Autodesk Inventor part; units mm, degrees
(part 2 of 4)
sketch "Sketch20" plane through (0, 0, 1.6) normal (0, 0, 1) x (1, 0, 0)
  line L0 (49, -24.373) -> (49, -33.5) projected
  arc A0 (47, -35.5) -> (49, -33.5) centre (47, -33.5) ccw projected
  line L1 (47, -35.5) -> (37, -35.5) projected
  arc A1 (35, -33.5) -> (37, -35.5) centre (37, -33.5) ccw projected
  line L2 (35, -33.5) -> (35, -24.373) projected
  arc A2 (37, -14.255) -> (35, -24.373) centre (42, -20.5) ccw projected
  line L3 (37, -14.255) -> (37, -6) projected
  arc A3 (47, -6) -> (37, -6) centre (42, -6) ccw projected
  line L4 (47, -6) -> (47, -14.255) projected
  arc A4 (49, -24.373) -> (47, -14.255) centre (42, -20.5) ccw projected
  line L5 (34.5, 22.1) -> (34.5, 39.1) projected
  arc A5 (35.5, 40.1) -> (34.5, 39.1) centre (35.5, 39.1) ccw projected
  line L6 (35.5, 40.1) -> (67.5, 40.1) projected
  arc A6 (68.5, 39.1) -> (67.5, 40.1) centre (67.5, 39.1) ccw projected
  line L7 (68.5, 39.1) -> (68.5, 22.1) projected
  arc A7 (67.5, 21.1) -> (68.5, 22.1) centre (67.5, 22.1) ccw projected
  line L8 (67.5, 21.1) -> (35.5, 21.1) projected
  arc A8 (34.5, 22.1) -> (35.5, 21.1) centre (35.5, 22.1) ccw projected
  circle A9 centre (35.75, 43.95) radius 3 projected
  circle A10 centre (67.25, 43.95) radius 3 projected
  circle A11 centre (67.25, 14.25) radius 3 projected
  circle A12 centre (35.75, 14.25) radius 3 projected
  circle A13 centre (-31.5, -14) radius 3.5 projected
  circle A14 centre (31.5, -14) radius 3.5 projected
  circle A15 centre (-10.5, -14) radius 3.5 projected
  circle A16 centre (10.5, -14) radius 3.5 projected
  line L9 (-47, -33.5) -> (-47, -26.745) projected
  arc A17 (-47, -14.255) -> (-47, -26.745) centre (-42, -20.5) ccw projected
  line L10 (-47, -14.255) -> (-47, -6) projected
  arc A18 (-37, -6) -> (-47, -6) centre (-42, -6) ccw projected
  line L11 (-37, -6) -> (-37, -14.255) projected
  arc A19 (-37, -26.745) -> (-37, -14.255) centre (-42, -20.5) ccw projected
  line L12 (-37, -26.745) -> (-37, -33.5) projected
  arc A20 (-39, -35.5) -> (-37, -33.5) centre (-39, -33.5) ccw projected
  line L13 (-39, -35.5) -> (-45, -35.5) projected
  arc A21 (-47, -33.5) -> (-45, -35.5) centre (-45, -33.5) ccw projected
  line L14 (-26, -33.5) -> (-26, -26.745) projected
  arc A22 (-26, -14.255) -> (-26, -26.745) centre (-21, -20.5) ccw projected
  line L15 (-26, -14.255) -> (-26, -6) projected
  arc A23 (-16, -6) -> (-26, -6) centre (-21, -6) ccw projected
  line L16 (-16, -6) -> (-16, -14.255) projected
  arc A24 (-16, -26.745) -> (-16, -14.255) centre (-21, -20.5) ccw projected
  line L17 (-16, -26.745) -> (-16, -33.5) projected
  arc A25 (-18, -35.5) -> (-16, -33.5) centre (-18, -33.5) ccw projected
  line L18 (-18, -35.5) -> (-24, -35.5) projected
  arc A26 (-26, -33.5) -> (-24, -35.5) centre (-24, -33.5) ccw projected
  line L19 (-5, -33.5) -> (-5, -26.745) projected
  arc A27 (-5, -14.255) -> (-5, -26.745) centre (0, -20.5) ccw projected
  line L20 (-5, -14.255) -> (-5, -6) projected
  arc A28 (5, -6) -> (-5, -6) centre (0, -6) ccw projected
  line L21 (5, -6) -> (5, -14.255) projected
  arc A29 (5, -26.745) -> (5, -14.255) centre (0, -20.5) ccw projected
  line L22 (5, -26.745) -> (5, -33.5) projected
  arc A30 (3, -35.5) -> (5, -33.5) centre (3, -33.5) ccw projected
  line L23 (3, -35.5) -> (-3, -35.5) projected
  arc A31 (-5, -33.5) -> (-3, -35.5) centre (-3, -33.5) ccw projected
  line L24 (16, -33.5) -> (16, -26.745) projected
  arc A32 (16, -14.255) -> (16, -26.745) centre (21, -20.5) ccw projected
  line L25 (16, -14.255) -> (16, -6) projected
  arc A33 (26, -6) -> (16, -6) centre (21, -6) ccw projected
  line L26 (26, -6) -> (26, -14.255) projected
  arc A34 (26, -26.745) -> (26, -14.255) centre (21, -20.5) ccw projected
  line L27 (26, -26.745) -> (26, -33.5) projected
  arc A35 (24, -35.5) -> (26, -33.5) centre (24, -33.5) ccw projected
  line L28 (24, -35.5) -> (18, -35.5) projected
  arc A36 (16, -33.5) -> (18, -35.5) centre (18, -33.5) ccw projected
  arc A37 (58, -6.5) -> (56, -8.5) centre (58, -8.5) ccw projected
  line L29 (58, -6.5) -> (70, -6.5) projected
  line L30 (70, -6.5) -> (70, -10.5) projected
  arc A38 (70, -10.5) -> (70.9655, -12.9138) centre (73.5, -10.5) ccw projected
  arc A39 (55.0345, -12.9138) -> (70.9655, -12.9138) centre (63, -20.5) ccw projected
  arc A40 (55.0345, -12.9138) -> (56, -10.5) centre (52.5, -10.5) ccw projected
  line L31 (56, -10.5) -> (56, -8.5) projected
  arc A41 (-58, -34.5) -> (-56, -32.5) centre (-58, -32.5) ccw projected
  line L32 (-58, -34.5) -> (-70, -34.5) projected
  line L33 (-70, -34.5) -> (-70, -30.5) projected
  arc A42 (-70, -30.5) -> (-70.9655, -28.0862) centre (-73.5, -30.5) ccw projected
  arc A43 (-55.0345, -28.0862) -> (-70.9655, -28.0862) centre (-63, -20.5) ccw projected
  arc A44 (-55.0345, -28.0862) -> (-56, -30.5) centre (-52.5, -30.5) ccw projected
  line L34 (-56, -30.5) -> (-56, -32.5) projected
  line L35 (-53.5, 10) -> (-68.5, 10) projected
  arc A45 (-70.7826, 16.1532) -> (-68.5, 10) centre (-68.5, 13.5) ccw projected
  arc A46 (-70.7826, 16.1532) -> (-70, 17.8589) centre (-72.25, 17.8589) ccw projected
  line L36 (-70, 17.8589) -> (-70, 22) projected
  line L37 (-70, 22) -> (-54, 22) projected
  arc A47 (-52, 20) -> (-54, 22) centre (-54, 20) ccw projected
  line L38 (-52, 20) -> (-52, 17.8589) projected
  arc A48 (-52, 17.8589) -> (-51.2174, 16.1532) centre (-49.75, 17.8589) ccw projected
  arc A49 (-53.5, 10) -> (-51.2174, 16.1532) centre (-53.5, 13.5) ccw projected
  line L39 (-70.5, -37.5) -> (-56.7679, -37.5) projected
  line L40 (-56.7679, -37.5) -> (-55.6132, -39.5) projected
  arc A50 (-55.6132, -41.5) -> (-55.6132, -39.5) centre (-57.3453, -40.5) ccw projected
  line L41 (-55.6132, -41.5) -> (-56.7679, -43.5) projected
  line L42 (-56.7679, -43.5) -> (-70.5, -43.5) projected
  line L43 (-70.5, -43.5) -> (-70.5, -47.4689) projected
  arc A51 (-70.5, -47.4689) -> (-69.0556, -48.3647) centre (-69.5, -47.4689) ccw projected
  arc A52 (-64.3647, -53.0556) -> (-69.0556, -48.3647) centre (-67.5, -51.5) ccw projected
  arc A53 (-64.3647, -53.0556) -> (-63.4689, -54.5) centre (-63.4689, -53.5) ccw projected
  line L44 (-63.4689, -54.5) -> (-47, -54.5) projected
  line L45 (-47, -54.5) -> (-47, -50) projected
  arc A54 (-45, -48) -> (-47, -50) centre (-45, -50) ccw projected
  line L46 (-45, -48) -> (24, -48) projected
  arc A55 (26, -50) -> (24, -48) centre (24, -50) ccw projected
  line L47 (26, -50) -> (26, -54.5) projected
  line L48 (26, -54.5) -> (63.4689, -54.5) projected
  arc A56 (63.4689, -54.5) -> (64.3647, -53.0556) centre (63.4689, -53.5) ccw projected
  arc A57 (69.0556, -48.3647) -> (64.3647, -53.0556) centre (67.5, -51.5) ccw projected
  arc A58 (69.0556, -48.3647) -> (70.5, -47.4689) centre (69.5, -47.4689) ccw projected
  line L49 (70.5, -47.4689) -> (70.5, -43.5) projected
  line L50 (70.5, -43.5) -> (57.2321, -43.5) projected
  line L51 (57.2321, -43.5) -> (58.5311, -41.25) projected
  arc A59 (58.5311, -41.25) -> (58.5311, -39.75) centre (57.2321, -40.5) ccw projected
  line L52 (58.5311, -39.75) -> (57.2321, -37.5) projected
  line L53 (57.2321, -37.5) -> (70.5, -37.5) projected
  line L54 (70.5, -37.5) -> (70.5, -30.5) projected
  arc A60 (71.3276, -28.431) -> (70.5, -30.5) centre (73.5, -30.5) ccw projected
  arc A61 (71.3276, -28.431) -> (71.3276, -12.569) centre (63, -20.5) ccw projected
  arc A62 (70.5, -10.5) -> (71.3276, -12.569) centre (73.5, -10.5) ccw projected
  line L55 (70.5, -10.5) -> (70.5, 9.6199) projected
  arc A63 (71, 10.9428) -> (70.5, 9.6199) centre (72.5, 9.6199) ccw projected
  arc A64 (71, 10.9428) -> (72.25, 14.25) centre (67.25, 14.25) ccw projected
  line L56 (72.25, 14.25) -> (72.25, 43.95) projected
  arc A65 (72.25, 43.95) -> (71, 47.2572) centre (67.25, 43.95) ccw projected
  arc A66 (70.6186, 47.9015) -> (71, 47.2572) centre (72.5, 48.5801) ccw projected
  arc A67 (70.6186, 47.9015) -> (69.194, 48.4372) centre (69.678, 47.5622) ccw projected
  arc A68 (64.3647, 53.0556) -> (69.194, 48.4372) centre (67.5, 51.5) ccw projected
  arc A69 (64.3647, 53.0556) -> (63.4689, 54.5) centre (63.4689, 53.5) ccw projected
  line L57 (63.4689, 54.5) -> (-63.4689, 54.5) projected
  arc A70 (-63.4689, 54.5) -> (-64.3647, 53.0556) centre (-63.4689, 53.5) ccw projected
  arc A71 (-69.0556, 48.3647) -> (-64.3647, 53.0556) centre (-67.5, 51.5) ccw projected
  arc A72 (-69.0556, 48.3647) -> (-70.5, 47.4689) centre (-69.5, 47.4689) ccw projected
  line L58 (-70.5, 47.4689) -> (-70.5, 17.8589) projected
  arc A73 (-71.1087, 16.5323) -> (-70.5, 17.8589) centre (-72.25, 17.8589) ccw projected
  arc A74 (-71.1087, 16.5323) -> (-71.1087, 10.4677) centre (-68.5, 13.5) ccw projected
  arc A75 (-70.5, 9.1411) -> (-71.1087, 10.4677) centre (-72.25, 9.1411) ccw projected
  line L59 (-70.5, 9.1411) -> (-70.5, 3) projected
  line L60 (-70.5, 3) -> (-53.1906, 3) projected
  line L61 (-53.1906, 3) -> (-51.7472, 0.5) projected
  arc A76 (-51.7472, -2.5) -> (-51.7472, 0.5) centre (-54.3453, -1) ccw projected
  line L62 (-51.7472, -2.5) -> (-53.1906, -5) projected
  line L63 (-53.1906, -5) -> (-70.5, -5) projected
  line L64 (-70.5, -5) -> (-70.5, -10.5) projected
  arc A77 (-71.3276, -12.569) -> (-70.5, -10.5) centre (-73.5, -10.5) ccw projected
  arc A78 (-71.3276, -12.569) -> (-71.3276, -28.431) centre (-63, -20.5) ccw projected
  arc A79 (-70.5, -30.5) -> (-71.3276, -28.431) centre (-73.5, -30.5) ccw projected
  line L65 (-70.5, -30.5) -> (-70.5, -37.5) projected
  line L66 (34, 39.1) -> (34, 22.1)
  arc A80 (34, 22.1) -> (35.5, 20.6) centre (35.5, 22.1) ccw
  line L67 (35.5, 20.6) -> (67.5, 20.6)
  arc A81 (67.5, 20.6) -> (69, 22.1) centre (67.5, 22.1) ccw
  line L68 (69, 22.1) -> (69, 39.1)
  arc A82 (69, 39.1) -> (67.5, 40.6) centre (67.5, 39.1) ccw
  line L69 (67.5, 40.6) -> (35.5, 40.6)
  arc A83 (35.5, 40.6) -> (34, 39.1) centre (35.5, 39.1) ccw
  line L70 (33.5, 39.1) -> (33.5, 22.1)
  arc A84 (33.5, 22.1) -> (35.5, 20.1) centre (35.5, 22.1) ccw
  line L71 (35.5, 20.1) -> (67.5, 20.1)
  arc A85 (67.5, 20.1) -> (69.5, 22.1) centre (67.5, 22.1) ccw
  line L72 (69.5, 22.1) -> (69.5, 39.1)
  arc A86 (69.5, 39.1) -> (67.5, 41.1) centre (67.5, 39.1) ccw
  line L73 (67.5, 41.1) -> (35.5, 41.1)
  arc A87 (35.5, 41.1) -> (33.5, 39.1) centre (35.5, 39.1) ccw
  circle A88 centre (35.75, 43.95) radius 4
  circle A89 centre (67.25, 43.95) radius 4
  line L74 (33, 22.1) -> (33, 39.1)
  arc A90 (35.5, 41.6) -> (33, 39.1) centre (35.5, 39.1) ccw
  line L75 (35.5, 41.6) -> (67.5, 41.6)
  arc A91 (70, 39.1) -> (67.5, 41.6) centre (67.5, 39.1) ccw
  line L76 (70, 39.1) -> (70, 22.1)
  arc A92 (67.5, 19.6) -> (70, 22.1) centre (67.5, 22.1) ccw
  line L77 (67.5, 19.6) -> (35.5, 19.6)
  arc A93 (33, 22.1) -> (35.5, 19.6) centre (35.5, 22.1) ccw
  line L78 (32.5, 22.1) -> (32.5, 39.1)
  arc A94 (35.5, 42.1) -> (32.5, 39.1) centre (35.5, 39.1) ccw
  line L79 (35.5, 42.1) -> (67.5, 42.1)
  arc A95 (70.5, 39.1) -> (67.5, 42.1) centre (67.5, 39.1) ccw
  line L80 (70.5, 39.1) -> (70.5, 22.1)
  arc A96 (67.5, 19.1) -> (70.5, 22.1) centre (67.5, 22.1) ccw
  line L81 (67.5, 19.1) -> (35.5, 19.1)
  arc A97 (32.5, 22.1) -> (35.5, 19.1) centre (35.5, 22.1) ccw
  point P0 (0, 0)
  point P1 (65.0643, 40.6)
  point P2 (64.4433, 41.1)
  point P3 (38.5567, 41.1)
  point P4 (37.9357, 40.6)
  point P5 (34.4469, 40.1682)
  point P6 (33.9581, 40.3738)
  point P7 (69.0419, 40.3738)
  point P8 (68.5531, 40.1682)
  point P9 (63.7035, 42.1)
  point P10 (39.2965, 42.1)
  point P11 (38.9869, 41.6)
  point P12 (64.0131, 41.6)
  point P13 (33.5215, 40.6283)
  point P14 (33.1245, 40.9322)
  point P15 (69.8755, 40.9322)
  point P16 (69.4785, 40.6283)
  dimension "d168" = 0.5
  dimension "d169" = 0.5
  dimension "d170" = 8
  dimension "d173" = 0.5
  dimension "d174" = 0.5
  constraints: 32 end point, 32 point on circle, 18 centre point, 2 coincident, 1 equal radius, 28 other
  measures "d168" distance between parallel lines of L5 L66
  measures "d169" distance between parallel lines of L72 L68
  measures "d170" diameter of A88
  measures "d173" distance between parallel lines of L80 L76
  measures "d174" distance between parallel lines of L76 L72
extrude "Extrusion15" add sketch "Sketch20" along normal up to surface (0.005 mm away) contours A83 L66 A80 L67 A81 L68 A82 A89 A86 L72 A85 L71 A84 L70 A87 A88 | A88 L73 A89 L69 | A90 L74 A93 L77 A92 L76 A91 A89 A95 L80 A96 L81 A97 L78 A94 A88 | A88 L79 A89 L75
sketch "Sketch23" plane through (42, -6, 1.605) normal (0, 0, 1) x (1, 0, 0)
  circle A0 centre (0, 0) radius 2.75 projected
  arc A1 (5, 0) -> (-5, 0) centre (0, 0) ccw projected
  line L0 (-5, -8.255) -> (-5, 0) projected
  arc A2 (5, -8.255) -> (-5, -8.255) centre (0, -14.5) ccw projected
  line L1 (5, 0) -> (5, -8.255) projected
  line L2 (0, 0) -> (0, -14.5) construction
  line L3 (-0.5, 0) -> (-0.5, -14.5)
  line L4 (0.5, -14.5) -> (0.5, 0)
  arc A3 (0.5, 0) -> (-0.5, 0) centre (0, 0) ccw
  arc A4 (-0.5, -14.5) -> (0.5, -14.5) centre (0, -14.5) ccw
  arc A5 (-0.5, -4.0389) -> (-1.4474, -2.3383) centre (-2.5, -4.0389) ccw
  arc A6 (1.4474, -2.3383) -> (0.5, -4.0389) centre (2.5, -4.0389) ccw
  circle A7 centre (0, 0) radius 2.75 projected
  line L5 (0, 0) -> (0, -24) construction
  line L6 (5, -29.5) -> (-5, -29.5) projected
  line L7 (4.5, 0) -> (4.5, -24)
  line L8 (-4.5, -24) -> (-4.5, 0)
  arc A8 (4.5, 0) -> (-4.5, 0) centre (0, 0) ccw
  arc A9 (-4.5, -24) -> (4.5, -24) centre (0, -24) ccw
  line L9 (-4, 0) -> (-4, -24)
  arc A10 (-4, -24) -> (4, -24) centre (0, -24) ccw
  line L10 (4, -24) -> (4, 0)
  arc A11 (4, 0) -> (-4, 0) centre (0, 0) ccw
  line L11 (-4.5, -24) -> (4.5, -24)
  arc A12 (-7, -18.373) -> (7, -18.373) centre (0, -14.5) ccw projected
  point P0 (-42, 6)
  point P1 (0, -7.25)
  point P2 (-0.5, -6.5156)
  point P3 (0.5, -6.5156)
  point P4 (0.5, -2.7042)
  point P5 (-0.5, -2.7042)
  point P6 (0, -12)
  point P7 (-4.5, -7.8856)
  point P8 (-4, -7.5718)
  point P9 (4, -7.5718)
  point P10 (4.5, -7.8856)
  point P11 (4.5, -21.1144)
  point P12 (4, -21.4282)
  point P13 (4, -24)
  point P14 (-4, -21.4282)
  point P15 (-4.5, -21.1144)
  point P16 (-4, -24)
  dimension "d188" = 1
  dimension "d189" = 2
  dimension "d192" = 0.5
  dimension "d193" = 0.5
  dimension "d194" = 5.5
  constraints: 22 end point, 18 point on circle, 12 tangent, 8 centre point, 3 parallel, 2 midpoint, 2 point on line, 1 equal radius, 1 horizontal, 1 perpendicular, 1 vertical, 3 other
  measures "d188" diameter of A4
  measures "d189" radius of A6
  measures "d192" radial gap between concentric circles of A8 A1
  measures "d193" radial gap between concentric circles of A11 A8
  measures "d194" distance between parallel lines of L6 L11
extrude "Extrusion18" add sketch "Sketch23" along normal up to surface (0.005 mm away) contours A2 L8 A8 L7 L10 A11 L9 | L9 L11 L8 A12 | A12 L7 L11 L10
sketch "Sketch24" plane through (0, 0, 1.6) normal (0, 0, 1) x (1, 0, 0)
  line L0 (33.5, 22.1) -> (33.5, 39.1) projected
  arc A0 (33.9581, 40.3738) -> (33.5, 39.1) centre (35.5, 39.1) ccw projected
  arc A1 (33.9581, 40.3738) -> (34.4469, 40.1682) centre (35.75, 43.95) ccw projected
  arc A2 (34.4469, 40.1682) -> (34, 39.1) centre (35.5, 39.1) ccw projected
  line L1 (34, 39.1) -> (34, 22.1) projected
  arc A3 (34, 22.1) -> (35.5, 20.6) centre (35.5, 22.1) ccw projected
  line L2 (35.5, 20.6) -> (67.5, 20.6) projected
  arc A4 (67.5, 20.6) -> (69, 22.1) centre (67.5, 22.1) ccw projected
  line L3 (69, 22.1) -> (69, 39.1) projected
  arc A5 (69, 39.1) -> (68.5531, 40.1682) centre (67.5, 39.1) ccw projected
  arc A6 (68.5531, 40.1682) -> (69.0419, 40.3738) centre (67.25, 43.95) ccw projected
  arc A7 (69.5, 39.1) -> (69.0419, 40.3738) centre (67.5, 39.1) ccw projected
  line L4 (69.5, 39.1) -> (69.5, 22.1) projected
  arc A8 (67.5, 20.1) -> (69.5, 22.1) centre (67.5, 22.1) ccw projected
  line L5 (67.5, 20.1) -> (35.5, 20.1) projected
  arc A9 (33.5, 22.1) -> (35.5, 20.1) centre (35.5, 22.1) ccw projected
  arc A10 (70.5, 39.1) -> (69.8755, 40.9322) centre (67.5, 39.1) ccw projected
  line L6 (70.5, 39.1) -> (70.5, 22.1) projected
  arc A11 (67.5, 19.1) -> (70.5, 22.1) centre (67.5, 22.1) ccw projected
  line L7 (67.5, 19.1) -> (35.5, 19.1) projected
  arc A12 (32.5, 22.1) -> (35.5, 19.1) centre (35.5, 22.1) ccw projected
  line L8 (32.5, 22.1) -> (32.5, 39.1) projected
  arc A13 (33.1245, 40.9322) -> (32.5, 39.1) centre (35.5, 39.1) ccw projected
  arc A14 (33.1245, 40.9322) -> (33.5215, 40.6283) centre (35.75, 43.95) ccw projected
  arc A15 (33.5215, 40.6283) -> (33, 39.1) centre (35.5, 39.1) ccw projected
  line L9 (33, 39.1) -> (33, 22.1) projected
  arc A16 (33, 22.1) -> (35.5, 19.6) centre (35.5, 22.1) ccw projected
  line L10 (35.5, 19.6) -> (67.5, 19.6) projected
  arc A17 (67.5, 19.6) -> (70, 22.1) centre (67.5, 22.1) ccw projected
  line L11 (70, 22.1) -> (70, 39.1) projected
  arc A18 (70, 39.1) -> (69.4785, 40.6283) centre (67.5, 39.1) ccw projected
  arc A19 (69.4785, 40.6283) -> (69.8755, 40.9322) centre (67.25, 43.95) ccw projected
  arc A20 (37.9357, 40.6) -> (38.5567, 41.1) centre (35.75, 43.95) ccw projected
  line L12 (38.5567, 41.1) -> (64.4433, 41.1) projected
  arc A21 (64.4433, 41.1) -> (65.0643, 40.6) centre (67.25, 43.95) ccw projected
  line L13 (65.0643, 40.6) -> (37.9357, 40.6) projected
  arc A22 (63.7035, 42.1) -> (64.0131, 41.6) centre (67.25, 43.95) ccw projected
  line L14 (64.0131, 41.6) -> (38.9869, 41.6) projected
  arc A23 (38.9869, 41.6) -> (39.2965, 42.1) centre (35.75, 43.95) ccw projected
  line L15 (39.2965, 42.1) -> (63.7035, 42.1) projected
  line L16 (49, -24.373) -> (49, -33.5) projected
  arc A24 (47, -35.5) -> (49, -33.5) centre (47, -33.5) ccw projected
  line L17 (47, -35.5) -> (37, -35.5) projected
  arc A25 (35, -33.5) -> (37, -35.5) centre (37, -33.5) ccw projected
  line L18 (35, -33.5) -> (35, -24.373) projected
  arc A26 (37, -14.255) -> (35, -24.373) centre (42, -20.5) ccw projected
  line L19 (37, -14.255) -> (37, -6) projected
  arc A27 (47, -6) -> (37, -6) centre (42, -6) ccw projected
  line L20 (47, -6) -> (47, -14.255) projected
  arc A28 (49, -24.373) -> (47, -14.255) centre (42, -20.5) ccw projected
  line L21 (34.5, 22.1) -> (34.5, 39.1) projected
  arc A29 (35.5, 40.1) -> (34.5, 39.1) centre (35.5, 39.1) ccw projected
  line L22 (35.5, 40.1) -> (67.5, 40.1) projected
  arc A30 (68.5, 39.1) -> (67.5, 40.1) centre (67.5, 39.1) ccw projected
  line L23 (68.5, 39.1) -> (68.5, 22.1) projected
  arc A31 (67.5, 21.1) -> (68.5, 22.1) centre (67.5, 22.1) ccw projected
  line L24 (67.5, 21.1) -> (35.5, 21.1) projected
  arc A32 (34.5, 22.1) -> (35.5, 21.1) centre (35.5, 22.1) ccw projected
  circle A33 centre (35.75, 43.95) radius 3 projected
  circle A34 centre (67.25, 43.95) radius 3 projected
  circle A35 centre (67.25, 14.25) radius 3 projected
  circle A36 centre (35.75, 14.25) radius 3 projected
  circle A37 centre (-31.5, -14) radius 3.5 projected
  circle A38 centre (31.5, -14) radius 3.5 projected
  circle A39 centre (-10.5, -14) radius 3.5 projected
  circle A40 centre (10.5, -14) radius 3.5 projected
  line L25 (-47, -33.5) -> (-47, -26.745) projected
  arc A41 (-47, -14.255) -> (-47, -26.745) centre (-42, -20.5) ccw projected
  line L26 (-47, -14.255) -> (-47, -6) projected
  arc A42 (-37, -6) -> (-47, -6) centre (-42, -6) ccw projected
  line L27 (-37, -6) -> (-37, -14.255) projected
  arc A43 (-37, -26.745) -> (-37, -14.255) centre (-42, -20.5) ccw projected
  line L28 (-37, -26.745) -> (-37, -33.5) projected
  arc A44 (-39, -35.5) -> (-37, -33.5) centre (-39, -33.5) ccw projected
  line L29 (-39, -35.5) -> (-45, -35.5) projected
  arc A45 (-47, -33.5) -> (-45, -35.5) centre (-45, -33.5) ccw projected
  line L30 (-26, -33.5) -> (-26, -26.745) projected
  arc A46 (-26, -14.255) -> (-26, -26.745) centre (-21, -20.5) ccw projected
  line L31 (-26, -14.255) -> (-26, -6) projected
  arc A47 (-16, -6) -> (-26, -6) centre (-21, -6) ccw projected
  line L32 (-16, -6) -> (-16, -14.255) projected
  arc A48 (-16, -26.745) -> (-16, -14.255) centre (-21, -20.5) ccw projected
  line L33 (-16, -26.745) -> (-16, -33.5) projected
  arc A49 (-18, -35.5) -> (-16, -33.5) centre (-18, -33.5) ccw projected
  line L34 (-18, -35.5) -> (-24, -35.5) projected
  arc A50 (-26, -33.5) -> (-24, -35.5) centre (-24, -33.5) ccw projected
  line L35 (-5, -33.5) -> (-5, -26.745) projected
  arc A51 (-5, -14.255) -> (-5, -26.745) centre (0, -20.5) ccw projected
  line L36 (-5, -14.255) -> (-5, -6) projected
  arc A52 (5, -6) -> (-5, -6) centre (0, -6) ccw projected
  line L37 (5, -6) -> (5, -14.255) projected
  arc A53 (5, -26.745) -> (5, -14.255) centre (0, -20.5) ccw projected
  line L38 (5, -26.745) -> (5, -33.5) projected
  arc A54 (3, -35.5) -> (5, -33.5) centre (3, -33.5) ccw projected
  line L39 (3, -35.5) -> (-3, -35.5) projected
  arc A55 (-5, -33.5) -> (-3, -35.5) centre (-3, -33.5) ccw projected
  line L40 (16, -33.5) -> (16, -26.745) projected
  arc A56 (16, -14.255) -> (16, -26.745) centre (21, -20.5) ccw projected
  line L41 (16, -14.255) -> (16, -6) projected
  arc A57 (26, -6) -> (16, -6) centre (21, -6) ccw projected
  line L42 (26, -6) -> (26, -14.255) projected
  arc A58 (26, -26.745) -> (26, -14.255) centre (21, -20.5) ccw projected
  line L43 (26, -26.745) -> (26, -33.5) projected
  arc A59 (24, -35.5) -> (26, -33.5) centre (24, -33.5) ccw projected
  line L44 (24, -35.5) -> (18, -35.5) projected
  arc A60 (16, -33.5) -> (18, -35.5) centre (18, -33.5) ccw projected
  arc A61 (58, -6.5) -> (56, -8.5) centre (58, -8.5) ccw projected
  line L45 (58, -6.5) -> (70, -6.5) projected
  line L46 (70, -6.5) -> (70, -10.5) projected
  arc A62 (70, -10.5) -> (70.9655, -12.9138) centre (73.5, -10.5) ccw projected
  arc A63 (55.0345, -12.9138) -> (70.9655, -12.9138) centre (63, -20.5) ccw projected
  arc A64 (55.0345, -12.9138) -> (56, -10.5) centre (52.5, -10.5) ccw projected
  line L47 (56, -10.5) -> (56, -8.5) projected
  arc A65 (-58, -34.5) -> (-56, -32.5) centre (-58, -32.5) ccw projected
  line L48 (-58, -34.5) -> (-70, -34.5) projected
  line L49 (-70, -34.5) -> (-70, -30.5) projected
  arc A66 (-70, -30.5) -> (-70.9655, -28.0862) centre (-73.5, -30.5) ccw projected
  arc A67 (-55.0345, -28.0862) -> (-70.9655, -28.0862) centre (-63, -20.5) ccw projected
  arc A68 (-55.0345, -28.0862) -> (-56, -30.5) centre (-52.5, -30.5) ccw projected
  line L50 (-56, -30.5) -> (-56, -32.5) projected
  line L51 (-53.5, 10) -> (-68.5, 10) projected
  arc A69 (-70.7826, 16.1532) -> (-68.5, 10) centre (-68.5, 13.5) ccw projected
  arc A70 (-70.7826, 16.1532) -> (-70, 17.8589) centre (-72.25, 17.8589) ccw projected
  line L52 (-70, 17.8589) -> (-70, 22) projected
  line L53 (-70, 22) -> (-54, 22) projected
  arc A71 (-52, 20) -> (-54, 22) centre (-54, 20) ccw projected
  line L54 (-52, 20) -> (-52, 17.8589) projected
  arc A72 (-52, 17.8589) -> (-51.2174, 16.1532) centre (-49.75, 17.8589) ccw projected
  arc A73 (-53.5, 10) -> (-51.2174, 16.1532) centre (-53.5, 13.5) ccw projected
  line L55 (-70.5, -37.5) -> (-56.7679, -37.5) projected
  line L56 (-56.7679, -37.5) -> (-55.6132, -39.5) projected
  arc A74 (-55.6132, -41.5) -> (-55.6132, -39.5) centre (-57.3453, -40.5) ccw projected
  line L57 (-55.6132, -41.5) -> (-56.7679, -43.5) projected
  line L58 (-56.7679, -43.5) -> (-70.5, -43.5) projected
  line L59 (-70.5, -43.5) -> (-70.5, -47.4689) projected
  arc A75 (-70.5, -47.4689) -> (-69.0556, -48.3647) centre (-69.5, -47.4689) ccw projected
  arc A76 (-64.3647, -53.0556) -> (-69.0556, -48.3647) centre (-67.5, -51.5) ccw projected
  arc A77 (-64.3647, -53.0556) -> (-63.4689, -54.5) centre (-63.4689, -53.5) ccw projected
  line L60 (-63.4689, -54.5) -> (-47, -54.5) projected
  line L61 (-47, -54.5) -> (-47, -50) projected
  arc A78 (-45, -48) -> (-47, -50) centre (-45, -50) ccw projected
  line L62 (-45, -48) -> (24, -48) projected
  arc A79 (26, -50) -> (24, -48) centre (24, -50) ccw projected
  line L63 (26, -50) -> (26, -54.5) projected
  line L64 (26, -54.5) -> (63.4689, -54.5) projected
  arc A80 (63.4689, -54.5) -> (64.3647, -53.0556) centre (63.4689, -53.5) ccw projected
  arc A81 (69.0556, -48.3647) -> (64.3647, -53.0556) centre (67.5, -51.5) ccw projected
  arc A82 (69.0556, -48.3647) -> (70.5, -47.4689) centre (69.5, -47.4689) ccw projected
  line L65 (70.5, -47.4689) -> (70.5, -43.5) projected
  line L66 (70.5, -43.5) -> (57.2321, -43.5) projected
  line L67 (57.2321, -43.5) -> (58.5311, -41.25) projected
  arc A83 (58.5311, -41.25) -> (58.5311, -39.75) centre (57.2321, -40.5) ccw projected
  line L68 (58.5311, -39.75) -> (57.2321, -37.5) projected
  line L69 (57.2321, -37.5) -> (70.5, -37.5) projected
  line L70 (70.5, -37.5) -> (70.5, -30.5) projected
  arc A84 (71.3276, -28.431) -> (70.5, -30.5) centre (73.5, -30.5) ccw projected
  arc A85 (71.3276, -28.431) -> (71.3276, -12.569) centre (63, -20.5) ccw projected
  arc A86 (70.5, -10.5) -> (71.3276, -12.569) centre (73.5, -10.5) ccw projected
  line L71 (70.5, -10.5) -> (70.5, 9.6199) projected
  arc A87 (71, 10.9428) -> (70.5, 9.6199) centre (72.5, 9.6199) ccw projected
  arc A88 (71, 10.9428) -> (72.25, 14.25) centre (67.25, 14.25) ccw projected
  line L72 (72.25, 14.25) -> (72.25, 43.95) projected
  arc A89 (72.25, 43.95) -> (71, 47.2572) centre (67.25, 43.95) ccw projected
  arc A90 (70.6186, 47.9015) -> (71, 47.2572) centre (72.5, 48.5801) ccw projected
  arc A91 (70.6186, 47.9015) -> (69.194, 48.4372) centre (69.678, 47.5622) ccw projected
  arc A92 (64.3647, 53.0556) -> (69.194, 48.4372) centre (67.5, 51.5) ccw projected
  arc A93 (64.3647, 53.0556) -> (63.4689, 54.5) centre (63.4689, 53.5) ccw projected
  line L73 (63.4689, 54.5) -> (-63.4689, 54.5) projected
  arc A94 (-63.4689, 54.5) -> (-64.3647, 53.0556) centre (-63.4689, 53.5) ccw projected
  arc A95 (-69.0556, 48.3647) -> (-64.3647, 53.0556) centre (-67.5, 51.5) ccw projected
  arc A96 (-69.0556, 48.3647) -> (-70.5, 47.4689) centre (-69.5, 47.4689) ccw projected
  line L74 (-70.5, 47.4689) -> (-70.5, 17.8589) projected
  arc A97 (-71.1087, 16.5323) -> (-70.5, 17.8589) centre (-72.25, 17.8589) ccw projected
  arc A98 (-71.1087, 16.5323) -> (-71.1087, 10.4677) centre (-68.5, 13.5) ccw projected
  arc A99 (-70.5, 9.1411) -> (-71.1087, 10.4677) centre (-72.25, 9.1411) ccw projected
  line L75 (-70.5, 9.1411) -> (-70.5, 3) projected
  line L76 (-70.5, 3) -> (-53.1906, 3) projected
  line L77 (-53.1906, 3) -> (-51.7472, 0.5) projected
  arc A100 (-51.7472, -2.5) -> (-51.7472, 0.5) centre (-54.3453, -1) ccw projected
  line L78 (-51.7472, -2.5) -> (-53.1906, -5) projected
  line L79 (-53.1906, -5) -> (-70.5, -5) projected
  line L80 (-70.5, -5) -> (-70.5, -10.5) projected
  arc A101 (-71.3276, -12.569) -> (-70.5, -10.5) centre (-73.5, -10.5) ccw projected
  arc A102 (-71.3276, -12.569) -> (-71.3276, -28.431) centre (-63, -20.5) ccw projected
  arc A103 (-70.5, -30.5) -> (-71.3276, -28.431) centre (-73.5, -30.5) ccw projected
  line L81 (-70.5, -30.5) -> (-70.5, -37.5) projected
  line L82 (-63.4689, 54) -> (63.4689, 54)
  arc A104 (63.9168, 53.2778) -> (63.4689, 54) centre (63.4689, 53.5) ccw
  arc A105 (63.9168, 53.2778) -> (69.436, 47.9997) centre (67.5, 51.5) ccw
  arc A106 (70.1483, 47.7318) -> (69.436, 47.9997) centre (69.678, 47.5622) ccw
  arc A107 (70.1483, 47.7318) -> (70.625, 46.9265) centre (72.5, 48.5801) ccw
  arc A108 (71.75, 43.95) -> (70.625, 46.9265) centre (67.25, 43.95) ccw
  line L83 (71.75, 43.95) -> (71.75, 14.25)
  arc A109 (70.625, 11.2735) -> (71.75, 14.25) centre (67.25, 14.25) ccw
  arc A110 (70.625, 11.2735) -> (70, 9.6199) centre (72.5, 9.6199) ccw
  line L84 (70, 9.6199) -> (70, -10.5)
  arc A111 (70, -10.5) -> (70.9655, -12.9138) centre (73.5, -10.5) ccw
  arc A112 (70.9655, -28.0862) -> (70.9655, -12.9138) centre (63, -20.5) ccw
  arc A113 (70.9655, -28.0862) -> (70, -30.5) centre (73.5, -30.5) ccw
  line L85 (70, -30.5) -> (70, -37)
  line L86 (70, -37) -> (56.366, -37)
  line L87 (56.366, -37) -> (58.0981, -40)
  arc A114 (58.0981, -41) -> (58.0981, -40) centre (57.2321, -40.5) ccw
  line L88 (58.0981, -41) -> (56.366, -44)
  line L89 (56.366, -44) -> (70, -44)
  line L90 (70, -44) -> (70, -47.4689)
  arc A115 (69.2778, -47.9168) -> (70, -47.4689) centre (69.5, -47.4689) ccw
  arc A116 (69.2778, -47.9168) -> (63.9168, -53.2778) centre (67.5, -51.5) ccw
  arc A117 (63.4689, -54) -> (63.9168, -53.2778) centre (63.4689, -53.5) ccw
  line L91 (63.4689, -54) -> (26.5, -54)
  line L92 (26.5, -54) -> (26.5, -50)
  arc A118 (26.5, -50) -> (24, -47.5) centre (24, -50) ccw
  line L93 (24, -47.5) -> (-45, -47.5)
  arc A119 (-45, -47.5) -> (-47.5, -50) centre (-45, -50) ccw
  line L94 (-47.5, -50) -> (-47.5, -54)
  line L95 (-47.5, -54) -> (-63.4689, -54)
  arc A120 (-63.9168, -53.2778) -> (-63.4689, -54) centre (-63.4689, -53.5) ccw
  arc A121 (-63.9168, -53.2778) -> (-69.2778, -47.9168) centre (-67.5, -51.5) ccw
  arc A122 (-70, -47.4689) -> (-69.2778, -47.9168) centre (-69.5, -47.4689) ccw
  line L96 (-70, -47.4689) -> (-70, -44)
  line L97 (-70, -44) -> (-56.4793, -44)
  line L98 (-56.4793, -44) -> (-55.1802, -41.75)
  arc A123 (-55.1802, -41.75) -> (-55.1802, -39.25) centre (-57.3453, -40.5) ccw
  line L99 (-55.1802, -39.25) -> (-56.4793, -37)
  line L100 (-56.4793, -37) -> (-70, -37)
  line L101 (-70, -37) -> (-70, -30.5)
  arc A124 (-70, -30.5) -> (-70.9655, -28.0862) centre (-73.5, -30.5) ccw
  arc A125 (-70.9655, -12.9138) -> (-70.9655, -28.0862) centre (-63, -20.5) ccw
  arc A126 (-70.9655, -12.9138) -> (-70, -10.5) centre (-73.5, -10.5) ccw
  line L102 (-70, -10.5) -> (-70, -5.5)
  line L103 (-70, -5.5) -> (-52.9019, -5.5)
  line L104 (-52.9019, -5.5) -> (-51.3142, -2.75)
  arc A127 (-51.3142, -2.75) -> (-51.3142, 0.75) centre (-54.3453, -1) ccw
  line L105 (-51.3142, 0.75) -> (-52.9019, 3.5)
  line L106 (-52.9019, 3.5) -> (-70, 3.5)
  line L107 (-70, 3.5) -> (-70, 9.1411)
  arc A128 (-70, 9.1411) -> (-70.7826, 10.8468) centre (-72.25, 9.1411) ccw
  arc A129 (-70.7826, 16.1532) -> (-70.7826, 10.8468) centre (-68.5, 13.5) ccw
  arc A130 (-70.7826, 16.1532) -> (-70, 17.8589) centre (-72.25, 17.8589) ccw
  line L108 (-70, 17.8589) -> (-70, 47.4689)
  arc A131 (-69.2778, 47.9168) -> (-70, 47.4689) centre (-69.5, 47.4689) ccw
  arc A132 (-69.2778, 47.9168) -> (-63.9168, 53.2778) centre (-67.5, 51.5) ccw
  arc A133 (-63.4689, 54) -> (-63.9168, 53.2778) centre (-63.4689, 53.5) ccw
  arc A134 (70.5, -10.5) -> (71.3276, -12.569) centre (73.5, -10.5) ccw
  line L109 (70.5, -10.5) -> (70.5, -6)
  line L110 (70.5, -6) -> (58, -6)
  arc A135 (58, -6) -> (55.5, -8.5) centre (58, -8.5) ccw
  line L111 (55.5, -8.5) -> (55.5, -10.5)
  arc A136 (54.6724, -12.569) -> (55.5, -10.5) centre (52.5, -10.5) ccw
  arc A137 (54.6724, -12.569) -> (71.3276, -12.569) centre (63, -20.5) ccw
  line L112 (47.5, -14.0193) -> (47.5, -6)
  arc A138 (47.5, -6) -> (36.5, -6) centre (42, -6) ccw
  line L113 (36.5, -6) -> (36.5, -14.0193)
  arc A139 (36.5, -14.0193) -> (34.5, -24.5) centre (42, -20.5) ccw
  line L114 (34.5, -24.5) -> (34.5, -33.5)
  arc A140 (34.5, -33.5) -> (37, -36) centre (37, -33.5) ccw
  line L115 (37, -36) -> (47, -36)
  arc A141 (47, -36) -> (49.5, -33.5) centre (47, -33.5) ccw
  line L116 (49.5, -33.5) -> (49.5, -24.5)
  arc A142 (49.5, -24.5) -> (47.5, -14.0193) centre (42, -20.5) ccw
  circle A143 centre (31.5, -14) radius 4
  line L117 (26.5, -14.0193) -> (26.5, -6)
  arc A144 (26.5, -6) -> (15.5, -6) centre (21, -6) ccw
  line L118 (15.5, -6) -> (15.5, -14.0193)
  arc A145 (15.5, -14.0193) -> (15.5, -26.9807) centre (21, -20.5) ccw
  line L119 (15.5, -26.9807) -> (15.5, -33.5)
  arc A146 (15.5, -33.5) -> (18, -36) centre (18, -33.5) ccw
  line L120 (18, -36) -> (24, -36)
  arc A147 (24, -36) -> (26.5, -33.5) centre (24, -33.5) ccw
  line L121 (26.5, -33.5) -> (26.5, -26.9807)
  arc A148 (26.5, -26.9807) -> (26.5, -14.0193) centre (21, -20.5) ccw
  line L122 (5.5, -14.0193) -> (5.5, -6)
  arc A149 (5.5, -6) -> (-5.5, -6) centre (0, -6) ccw
  line L123 (-5.5, -6) -> (-5.5, -14.0193)
  arc A150 (-5.5, -14.0193) -> (-5.5, -26.9807) centre (0, -20.5) ccw
  line L124 (-5.5, -26.9807) -> (-5.5, -33.5)
  arc A151 (-5.5, -33.5) -> (-3, -36) centre (-3, -33.5) ccw
  line L125 (-3, -36) -> (3, -36)
  arc A152 (3, -36) -> (5.5, -33.5) centre (3, -33.5) ccw
  line L126 (5.5, -33.5) -> (5.5, -26.9807)
  arc A153 (5.5, -26.9807) -> (5.5, -14.0193) centre (0, -20.5) ccw
  circle A154 centre (10.5, -14) radius 4
  circle A155 centre (-10.5, -14) radius 4
  line L127 (-15.5, -14.0193) -> (-15.5, -6)
  arc A156 (-15.5, -6) -> (-26.5, -6) centre (-21, -6) ccw
  line L128 (-26.5, -6) -> (-26.5, -14.0193)
  arc A157 (-26.5, -14.0193) -> (-26.5, -26.9807) centre (-21, -20.5) ccw
  line L129 (-26.5, -26.9807) -> (-26.5, -33.5)
  arc A158 (-26.5, -33.5) -> (-24, -36) centre (-24, -33.5) ccw
  line L130 (-24, -36) -> (-18, -36)
  arc A159 (-18, -36) -> (-15.5, -33.5) centre (-18, -33.5) ccw
  line L131 (-15.5, -33.5) -> (-15.5, -26.9807)
  arc A160 (-15.5, -26.9807) -> (-15.5, -14.0193) centre (-21, -20.5) ccw
  circle A161 centre (-31.5, -14) radius 4
  line L132 (-36.5, -14.0193) -> (-36.5, -6)
  arc A162 (-36.5, -6) -> (-47.5, -6) centre (-42, -6) ccw
  line L133 (-47.5, -6) -> (-47.5, -14.0193)
  arc A163 (-47.5, -14.0193) -> (-47.5, -26.9807) centre (-42, -20.5) ccw
  line L134 (-47.5, -26.9807) -> (-47.5, -33.5)
  arc A164 (-47.5, -33.5) -> (-45, -36) centre (-45, -33.5) ccw
  line L135 (-45, -36) -> (-39, -36)
  arc A165 (-39, -36) -> (-36.5, -33.5) centre (-39, -33.5) ccw
  line L136 (-36.5, -33.5) -> (-36.5, -26.9807)
  arc A166 (-36.5, -26.9807) -> (-36.5, -14.0193) centre (-42, -20.5) ccw
  arc A167 (-70.5, -30.5) -> (-71.3276, -28.431) centre (-73.5, -30.5) ccw
  line L137 (-70.5, -30.5) -> (-70.5, -35)
  line L138 (-70.5, -35) -> (-58, -35)
  arc A168 (-58, -35) -> (-55.5, -32.5) centre (-58, -32.5) ccw
  line L139 (-55.5, -32.5) -> (-55.5, -30.5)
  arc A169 (-54.6724, -28.431) -> (-55.5, -30.5) centre (-52.5, -30.5) ccw
  arc A170 (-54.6724, -28.431) -> (-71.3276, -28.431) centre (-63, -20.5) ccw
  line L140 (-54, 22.5) -> (-70.5, 22.5)
  line L141 (-70.5, 22.5) -> (-70.5, 17.8589)
  arc A171 (-71.1087, 16.5323) -> (-70.5, 17.8589) centre (-72.25, 17.8589) ccw
  arc A172 (-71.1087, 16.5323) -> (-68.5, 9.5) centre (-68.5, 13.5) ccw
  line L142 (-68.5, 9.5) -> (-53.5, 9.5)
  arc A173 (-53.5, 9.5) -> (-50.8913, 16.5323) centre (-53.5, 13.5) ccw
  arc A174 (-51.5, 17.8589) -> (-50.8913, 16.5323) centre (-49.75, 17.8589) ccw
  line L143 (-51.5, 17.8589) -> (-51.5, 20)
  arc A175 (-51.5, 20) -> (-54, 22.5) centre (-54, 20) ccw
  line L144 (32, 39.1) -> (32, 22.1)
  arc A176 (32, 22.1) -> (35.5, 18.6) centre (35.5, 22.1) ccw
  line L145 (35.5, 18.6) -> (67.5, 18.6)
  arc A177 (67.5, 18.6) -> (71, 22.1) centre (67.5, 22.1) ccw
  line L146 (71, 22.1) -> (71, 39.1)
  arc A178 (71, 39.1) -> (67.5, 42.6) centre (67.5, 39.1) ccw
  line L147 (67.5, 42.6) -> (35.5, 42.6)
  arc A179 (35.5, 42.6) -> (32, 39.1) centre (35.5, 39.1) ccw
  point P0 (0, 0)
  point P1 (-70, 22.5)
  point P2 (-70.1109, 9.8387)
  point P3 (-70.1419, -11.4865)
  point P4 (-70, -35)
  point P5 (70.1419, -29.5135)
  point P6 (70, -6)
  point P7 (34.3389, -16.8179)
  point P8 (28.6611, -16.8179)
  point P9 (13.3389, -16.8179)
  point P10 (7.6611, -16.8179)
  point P11 (-7.6611, -16.8179)
  point P12 (-13.3389, -16.8179)
  point P13 (-28.6611, -16.8179)
  point P14 (-34.3389, -16.8179)
  point P15 (-35.2881, -15.2846)
  point P16 (-27.7119, -15.2846)
  point P17 (-14.2881, -15.2846)
  point P18 (-6.7119, -15.2846)
  point P19 (6.7119, -15.2846)
  point P20 (14.2881, -15.2846)
  point P21 (27.7119, -15.2846)
  point P22 (35.2881, -15.2846)
  point P23 (33.4964, 41.9698)
  point P24 (38.4291, 42.6)
  point P25 (64.5709, 42.6)
  point P26 (69.5036, 41.9698)
  dimension "d195" = 0.5
  dimension "d196" = 0.5
  dimension "d197" = 0.5
  dimension "d198" = 0.5
  dimension "d199" = 0.5
  dimension "d200" = 0.5
  dimension "d201" = 0.5
  dimension "d202" = 0.5
  dimension "d203" = 0.5
  dimension "d204" = 0.5
  dimension "d205" = 0.5
  dimension "d206" = 0.5
  dimension "d207" = 0.5
  dimension "d208" = 0.5
  constraints: 144 point on circle, 132 end point, 76 centre point, 128 other
  measures "d195" distance between parallel lines of L73 L82
  measures "d196" radial gap between concentric circles of A63 A137
  measures "d197" distance between parallel lines of L20 L112
  measures "d198" radial gap between concentric circles of A38 A143
  measures "d199" distance between parallel lines of L42 L117
  measures "d200" radial gap between concentric circles of A53 A153
  measures "d201" radial gap between concentric circles of A40 A154
  measures "d202" radial gap between concentric circles of A39 A155
  measures "d203" distance between parallel lines of L32 L127
  measures "d204" radial gap between concentric circles of A37 A161
  measures "d205" distance between parallel lines of L27 L132
  measures "d206" radial gap between concentric circles of A67 A170
  measures "d207" radial gap between concentric circles of A71 A175
  measures "d208" distance between parallel lines of L144 L8
extrude "Extrusion19" add sketch "Sketch24" along normal blind 0.2 contours L110 A135 L111 A136 A137 A113 L85 L86 L87 A114 L88 L89 L90 A115 A116 A117 L91 L92 A118 L93 A119 L94 L95 A120 A121 A122 L96 L97 L98 A123 L99 L100 L101 L138 A168 L139 A169 A170 A126 L102 L103 L104 A127 L105 L106 L107 A128 A172 L142 A173 A174 L143 A175 L140 L108 A131 A132 A133 L82 A104 A105 A106 A107 A108 L83 A109 A110 L84